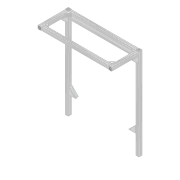
# Autodesk Inventor part: item_2019-08-21_Engineering_Project_Projekt_ID-1d05e1fc38aaeca349
Saved by Autodesk Inventor 2019 (Build 230136000, 136)
## iProperties
Created: 2019-10-22
Part Number: item_2019-08-21_Engineering_Project_Projekt_ID-1d05e1fc38aaeca349
Material: Generic
Document SubType Name: Modeling
Designer: romanp
Density: 1 g/cm^3
Appearance: Default
Author: romanp
Autodesk Inventor part; units mm, degrees
ref_plane "YZ Plane" through (0, 0, 0) normal (1, 0, 0) x (0, 1, 0)
ref_plane "XZ Plane" through (0, 0, 0) normal (0, 1, 0) x (-1, 0, 0)
ref_plane "XY Plane" through (0, 0, 0) normal (0, 0, 1) x (1, 0, 0)
sketch "Sketch2" plane through (-1413.3499, -32.973, 86.765) normal (0, 1, 0) x (-1, 0, 0)
  circle A0 centre (-482.0015, 2.6031) radius 3
  circle A1 centre (-512.0015, 2.6031) radius 3
  point P0 (-1413.3499, -86.765)
  dimension "d11" = 6
  dimension "d12" = 6
  constraints: 2 centre point
  measures "d11" diameter of A0
  measures "d12" diameter of A1
extrude "Extrusion1" add sketch "Sketch2" against normal blind 40
body "Solid1"
